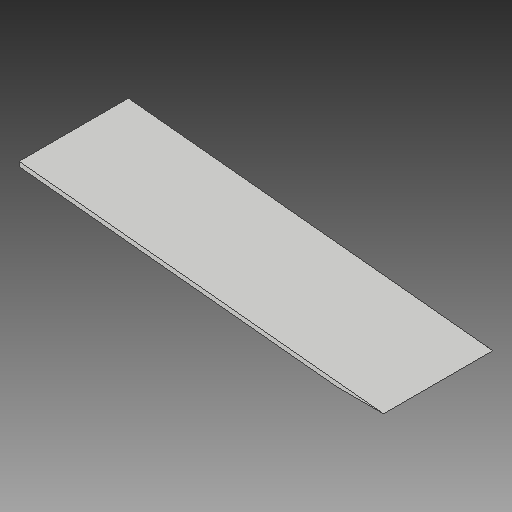
# Autodesk Inventor part: Ramp1
Saved by Autodesk Inventor 2019 (Build 230136000, 136)
## iProperties
Created: 2018-09-21
Part Number: Ramp1
Material: Generic
Document SubType Name: Modeling
Designer: user
Density: 1 g/cm^3
Appearance: Default
Author: user
Autodesk Inventor part; units mm, degrees
ref_plane "YZ Plane" through (0, 0, 0) normal (1, 0, 0) x (0, 1, 0)
ref_plane "XZ Plane" through (0, 0, 0) normal (0, 1, 0) x (-1, 0, 0)
ref_plane "XY Plane" through (0, 0, 0) normal (0, 0, 1) x (1, 0, 0)
sketch "Sketch1" plane through (0, 0, 0) normal (0, 0, 1) x (1, 0, 0)
  line L0 (457.2, 0) -> (457.2, 19.05) projected
  line L1 (457.2, -133.35) -> (457.2, 0) projected
  line L2 (0, 0) -> (0, -133.35) projected
  line L3 (457.2, 19.05) -> (1981.2, -133.35)
  line L4 (1789.7499, -133.35) -> (457.2, -0.095)
  line L5 (1789.7499, -133.35) -> (1981.2, -133.35)
  dimension "d3" = 19.05
  dimension "d4" = 1981.2
  constraints: 6 end point, 1 horizontal, 1 horizontal alignment, 1 parallel, 1 point on line
  measures "d3" distance between parallel lines of L3 L4
  measures "d4" distance from line of L3.end L2
extrude "Extrusion1" add sketch "Sketch1" against normal blind 457.2
body "Solid1"
